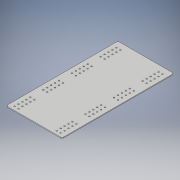
# Autodesk Inventor part: Plastic Inlay
Saved by Autodesk Inventor 2019.4 (Build 234330000, 330)
## iProperties
Created: 2021-04-06
Part Number: Plastic Inlay
Material: Generic
Document SubType Name: Modeling
Designer: caleb
Density: 1 g/cm^3
Appearance: Default
Author: caleb
Autodesk Inventor part; units mm, degrees
ref_plane "YZ Plane" through (0, 0, 0) normal (1, 0, 0) x (0, 1, 0)
ref_plane "XZ Plane" through (0, 0, 0) normal (0, 1, 0) x (-1, 0, 0)
ref_plane "XY Plane" through (0, 0, 0) normal (0, 0, 1) x (1, 0, 0)
sketch "Sketch1" plane through (0, 0, 0) normal (0, 1, 0) x (-1, 0, 0)
  line L0 (-50.8, 101.6) -> (50.8, 101.6)
  line L1 (50.8, 101.6) -> (50.8, -101.6)
  line L2 (50.8, -101.6) -> (-50.8, -101.6)
  line L3 (-50.8, -101.6) -> (-50.8, 101.6)
  line L4 (-50.8, 101.6) -> (50.8, -101.6) construction
  line L5 (50.8, 101.6) -> (-50.8, -101.6) construction
  point P0 (0, 0)
  dimension "d0" = 101.6
  dimension "d1" = 203.2
  constraints: 12 end point, 2 midpoint, 2 parallel, 1 horizontal, 1 perpendicular
  measures "d0" distance of L1.end L2.end
  measures "d1" distance of L0.end L1.end
extrude "Extrusion1" add sketch "Sketch1" along normal blind 1.5875
sketch "Sketch2" plane through (0, 1.5875, 0) normal (0, 1, 0) x (1, 0, 0)
  line L0 (-50.8, 101.6) -> (-50.8, -101.6) projected
  line L1 (-50.8, -101.6) -> (50.8, -101.6) projected
  line L2 (50.8, -101.6) -> (50.8, 101.6) projected
  point P0 (0, 0)
  point P1 (-41.91, -95.25)
  point P2 (-41.91, -88.1062)
  point P3 (-41.91, -80.9625)
  point P4 (-41.91, -73.8187)
  point P5 (-41.91, -66.675)
  point P6 (-34.7662, -95.25)
  point P7 (-34.7662, -88.1062)
  point P8 (-34.7662, -80.9625)
  point P9 (-34.7662, -73.8187)
  point P10 (-34.7662, -66.675)
  point P11 (-41.91, -43.053)
  point P12 (-34.7663, -43.053)
  point P13 (-34.7663, -35.9092)
  point P14 (-41.91, -35.9092)
  point P15 (-41.91, -28.7655)
  point P16 (-34.7663, -28.7655)
  point P17 (-34.7663, -21.6217)
  point P18 (-34.7663, -14.478)
  point P19 (-41.91, -14.478)
  point P20 (-41.91, -21.6217)
  point P21 (-41.91, 9.144)
  point P22 (-34.7663, 9.144)
  point P23 (-34.7663, 16.2878)
  point P24 (-41.91, 16.2878)
  point P25 (-41.91, 23.4315)
  point P26 (-34.7663, 23.4315)
  point P27 (-34.7663, 30.5753)
  point P28 (-34.7663, 37.719)
  point P29 (-41.91, 37.719)
  point P30 (-41.91, 30.5753)
  point P31 (-41.91, 61.341)
  point P32 (-34.7663, 61.341)
  point P33 (-34.7663, 68.4848)
  point P34 (-41.91, 68.4848)
  point P35 (-41.91, 75.6285)
  point P36 (-34.7663, 75.6285)
  point P37 (-34.7663, 82.7723)
  point P38 (-34.7663, 89.916)
  point P39 (-41.91, 89.916)
  point P40 (-41.91, 82.7723)
  point P41 (34.7599, -95.25)
  point P42 (41.9036, -95.25)
  point P43 (41.9036, -88.1063)
  point P44 (34.7599, -88.1063)
  point P45 (34.7599, -80.9625)
  point P46 (41.9036, -80.9625)
  point P47 (41.9036, -73.8187)
  point P48 (41.9036, -66.675)
  point P49 (34.7599, -66.675)
  point P50 (34.7599, -73.8187)
  point P51 (34.7599, -43.053)
  point P52 (41.9036, -43.053)
  point P53 (41.9036, -35.9092)
  point P54 (34.7599, -35.9092)
  point P55 (34.7599, -28.7655)
  point P56 (41.9036, -28.7655)
  point P57 (41.9036, -21.6217)
  point P58 (41.9036, -14.478)
  point P59 (34.7599, -14.478)
  point P60 (34.7599, -21.6217)
  point P61 (34.7599, 9.144)
  point P62 (41.9036, 9.144)
  point P63 (41.9036, 16.2878)
  point P64 (34.7599, 16.2878)
  point P65 (34.7599, 23.4315)
  point P66 (41.9036, 23.4315)
  point P67 (41.9036, 30.5753)
  point P68 (41.9036, 37.719)
  point P69 (34.7599, 37.719)
  point P70 (34.7599, 30.5753)
  point P71 (34.7599, 61.341)
  point P72 (41.9036, 61.341)
  point P73 (41.9036, 68.4848)
  point P74 (34.7599, 68.4848)
  point P75 (34.7599, 75.6285)
  point P76 (41.9036, 75.6285)
  point P77 (41.9036, 82.7723)
  point P78 (41.9036, 89.916)
  point P79 (34.7599, 89.916)
  point P80 (34.7599, 82.7723)
  dimension "d4" = 8.89
  dimension "d5" = 6.35
  dimension "d8" = 7.1437
  dimension "d11" = 7.1437
  dimension "d23" = 52.197
  dimension "d26" = 76.6699
  dimension "d30" = 8.8963
  constraints: 2 horizontal, 2 vertical, 79 other
  measures "d4" distance from line of L0 point (-41.91, -95.25)
  measures "d5" distance from line of L1 point (-41.91, -95.25)
  measures "d8" distance of point (-41.91, -95.25) point (-41.91, -88.106)
  measures "d11" distance of point (-41.91, -95.25) point (-34.766, -95.25)
  measures "d23" distance of point (-41.91, -95.25) point (-41.91, -43.053)
  measures "d26" distance of point (-41.91, -95.25) point (34.76, -95.25)
  measures "d30" distance from line of L2 point (41.904, -95.25)
hole "Hole1" at (-41.91, 1.5875, 95.25) at (-41.91, 1.5875, 88.1062) at (-41.91, 1.5875, 80.9625) at (-41.91, 1.5875, 73.8187) at (-41.91, 1.5875, 66.675) at (-34.7662, 1.5875, 95.25) at (-34.7662, 1.5875, 88.1062) at (-34.7662, 1.5875, 80.9625) at (-34.7662, 1.5875, 73.8187) at (-34.7662, 1.5875, 66.675) at (-41.91, 1.5875, 43.053) at (-34.7663, 1.5875, 43.053) at (-34.7663, 1.5875, 35.9092) at (-41.91, 1.5875, 35.9092) at (-34.7663, 1.5875, 28.7655) at (-41.91, 1.5875, 28.7655) at (-34.7663, 1.5875, 21.6217) at (-41.91, 1.5875, 21.6217) at (-34.7663, 1.5875, 14.478) at (-41.91, 1.5875, 14.478) at (-34.7663, 1.5875, -37.719) at (-41.91, 1.5875, -37.719) at (-41.91, 1.5875, -30.5753) at (-34.7663, 1.5875, -30.5753) at (-34.7663, 1.5875, -23.4315) at (-41.91, 1.5875, -23.4315) at (-34.7663, 1.5875, -16.2878) at (-41.91, 1.5875, -16.2878) at (-41.91, 1.5875, -9.144) at (-34.7663, 1.5875, -9.144) at (-34.7663, 1.5875, -61.341) at (-34.7663, 1.5875, -68.4848) at (-34.7663, 1.5875, -75.6285) at (-34.7663, 1.5875, -82.7723) at (-34.7663, 1.5875, -89.916) at (-41.91, 1.5875, -89.916) at (-41.91, 1.5875, -82.7723) at (-41.91, 1.5875, -75.6285) at (-41.91, 1.5875, -68.4848) at (-41.91, 1.5875, -61.341) at (41.9036, 1.5875, -89.916) at (34.7599, 1.5875, -89.916) at (41.9036, 1.5875, -82.7723) at (34.7599, 1.5875, -82.7723) at (41.9036, 1.5875, -75.6285) at (34.7599, 1.5875, -75.6285) at (41.9036, 1.5875, -68.4848) at (34.7599, 1.5875, -68.4848) at (41.9036, 1.5875, -61.341) at (34.7599, 1.5875, -61.341) direction (0, -1, 0) diameter 2.3813 end through all and at (41.9036, 1.5875, -37.719) (34.7599, 1.5875, -37.719) (34.7599, 1.5875, -30.5753) (41.9036, 1.5875, -30.5753) (41.9036, 1.5875, -23.4315) (34.7599, 1.5875, -23.4315) (34.7599, 1.5875, -16.2878) (41.9036, 1.5875, -16.2878) (41.9036, 1.5875, -9.144) (34.7599, 1.5875, -9.144) (41.9036, 1.5875, 14.478) (34.7599, 1.5875, 14.478) (34.7599, 1.5875, 21.6217) (41.9036, 1.5875, 21.6217) (41.9036, 1.5875, 28.7655) (34.7599, 1.5875, 28.7655) (34.7599, 1.5875, 35.9092) (41.9036, 1.5875, 35.9092) (41.9036, 1.5875, 43.053) (34.7599, 1.5875, 43.053) (41.9036, 1.5875, 66.675) (41.9036, 1.5875, 73.8187) (41.9036, 1.5875, 80.9625) (41.9036, 1.5875, 88.1063) (41.9036, 1.5875, 95.25) (34.7599, 1.5875, 95.25) (34.7599, 1.5875, 88.1063) (34.7599, 1.5875, 80.9625) (34.7599, 1.5875, 73.8187) (34.7599, 1.5875, 66.675)
fillet "Fillet1" radius 3.175 4 edges at (-50.8, 0.7937, 101.6) (-50.8, 0.7937, -101.6) (50.8, 0.7937, -101.6) (50.8, 0.7937, 101.6)
body "Solid1"
